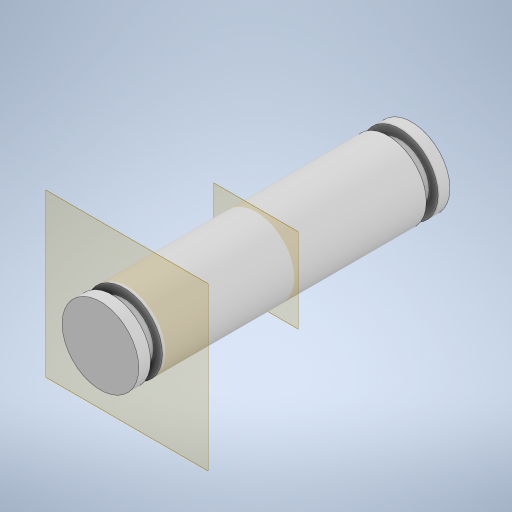
# Autodesk Inventor part: axle-middle
Saved by Autodesk Inventor 2024 (Build 280153000, 153)
## iProperties
Created: 2024-04-10
Part Number: axle-middle
Material: Generic
Document SubType Name: Modeling
Designer: MaartenGeorgesBuelen
Density: 1 g/cm^3
Appearance: Default
Author: MaartenGeorgesBuelen
## iProperties of the stored document axle-middle_3DPrint.ipt
Created: 2024-04-10
Part Number: axle-middle_3DPrint
Material: Generic
Document SubType Name: Modeling
Designer: MaartenGeorgesBuelen
Density: 1 g/cm^3
Appearance: Default
Author: MaartenGeorgesBuelen
Autodesk Inventor part; units mm, degrees
ref_plane "YZ Plane" through (0, 0, 0) normal (1, 0, 0) x (0, 1, 0)
ref_plane "XZ Plane" through (0, 0, 0) normal (0, 1, 0) x (-1, 0, 0)
ref_plane "Work Plane1" through (0, 0, 0) normal (0, 0, 1) x (1, 0, 0)
sketch "Sketch1" plane through (0, 0, 0) normal (0, 0, 1) x (1, 0, 0)
  circle A0 centre (0, 0) radius 13.5 projected
  circle A1 centre (0, 0) radius 13
  point P0 (0, 0)
  dimension "d0" = 0.5
  constraints: 1 centre point
  measures "d0" radial gap between concentric circles of A0 A1
ref_plane "Work Plane2" through (-25, -25, -87.5) normal (0, 0, -1) x (0, 1, 0)
extrude "Extrusion1" add sketch "Sketch1" against normal up to surface (87.5 mm away) contours A1
move faces "Move1" translate (0, 0, -1) faces at (3.1176, -1.8365, -87.5)
move faces "Move2" translate (0, 0, 1) faces at (3.1176, -1.8365, 0)
sketch "Sketch3" plane through (0, 0, 1) normal (0, 0, 1) x (1, 0, 0)
  circle A0 centre (0, 0) radius 10
  dimension "d11" = 20
  constraints: 1 centre point, 1 coincident
  measures "d11" diameter of A0
extrude "Extrusion3" add sketch "Sketch3" along normal blind 4
sketch "Sketch4" plane through (0, 0, 5) normal (0, 0, 1) x (1, 0, 0)
  circle A0 centre (0, 0) radius 10 projected
  circle A1 centre (0, 0) radius 13 projected
extrude "Extrusion4" add sketch "Sketch4" along normal blind 4 contours A0 | A1
ref_plane "Work Plane3" through (0, 0, -43.75) normal (0, 0, 1) x (1, 0, 0)
mirror "Mirror1" about plane through (0, 0, -43.75) normal (0, 0, 1) of "Extrusion3", "Extrusion4"
body "Solid1"
